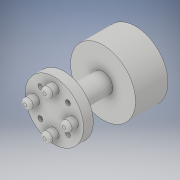
# Autodesk Inventor part: Motor1Gear
Saved by Autodesk Inventor 2019 (Build 230136000, 136)
## iProperties
Created: 2022-08-23
Part Number: Motor1Gear
Material: Generic
Document SubType Name: Modeling
Designer: zreik
Density: 1 g/cm^3
Appearance: Default
Author: zreik
Autodesk Inventor part; units mm, degrees
ref_plane "YZ Plane" through (0, 0, 0) normal (1, 0, 0) x (0, 1, 0)
ref_plane "XZ Plane" through (0, 0, 0) normal (0, 1, 0) x (-1, 0, 0)
ref_plane "XY Plane" through (0, 0, 0) normal (0, 0, 1) x (1, 0, 0)
sketch "Sketch1" plane through (0, 0, 0) normal (0, 0, 1) x (1, 0, 0)
  circle A0 centre (0, 0) radius 10
  dimension "d0" = 20
  constraints: 1 centre point, 1 coincident
  measures "d0" diameter of A0
extrude "Extrusion1" add sketch "Sketch1" along normal blind 10
sketch "Sketch2" plane through (0, 0, 10) normal (0, 0, 1) x (1, 0, 0)
  circle A0 centre (0, 0) radius 3
  dimension "d3" = 6
  constraints: 1 centre point, 1 coincident
  measures "d3" diameter of A0
extrude "Extrusion2" add sketch "Sketch2" along normal blind 12
sketch "Sketch3" plane through (0, 0, 22) normal (0, 0, 1) x (1, 0, 0)
  circle A0 centre (0, 0) radius 9
  dimension "d6" = 18
  constraints: 1 centre point, 1 coincident
  measures "d6" diameter of A0
extrude "Extrusion3" add sketch "Sketch3" along normal blind 3
sketch "Sketch4" plane through (0, 0, 25) normal (0, 0, 1) x (1, 0, 0)
  circle A0 centre (0, 6) radius 1.5
  circle A1 centre (4.2426, 4.2426) radius 0.75
  line L0 (0, 0) -> (0, 14.9818) construction
  line L1 (0, 0) -> (4.2426, 4.2426) construction
  dimension "d9" = 3
  dimension "d10" = 1.5
  dimension "d11" = 0
  dimension "d12" = 6
  dimension "d13" = 45
  dimension "d14" = 0
  dimension "d15" = 6
  dimension "d16" = 0
  constraints: 4 end point, 2 centre point, 1 vertical
  measures "d9" diameter of A0
  measures "d10" diameter of A1
  measures "d11" horizontal distance of L0.start A0.centre
  measures "d12" distance of L0.start A0.centre
  measures "d13" angle of L1 L0
  measures "d14" distance from line of L1 A1.centre
  measures "d15" distance of L0.start L1.end
  measures "d16" distance of L1.end A1.centre
extrude "Extrusion4" add sketch "Sketch4" along normal blind 3 contours A0
extrude "Extrusion5" cut sketch "Sketch4" against normal blind 3 contours A1
fillet "Fillet1" radius 1 1 edges at (-1.5, 6, 28)
pattern_circular "Circular Pattern1" count 4 over 360 about axis through (0, 0, 22) along (0, 0, 1) of "Extrusion4", "Fillet1", "Extrusion5"
body "Solid1"
